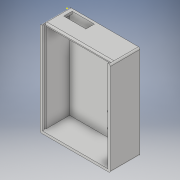
# Autodesk Inventor part: BatteryBox
Saved by Autodesk Inventor 2019 (Build 230136000, 136)
## iProperties
Created: 2018-06-02
Part Number: BatteryBox
Material: Generic
Document SubType Name: Modeling
Designer: samps
Density: 1 g/cm^3
Appearance: Default
Author: samps
Autodesk Inventor part; units mm, degrees
ref_plane "YZ Plane" through (0, 0, 0) normal (1, 0, 0) x (0, 1, 0)
ref_plane "XZ Plane" through (0, 0, 0) normal (0, 1, 0) x (-1, 0, 0)
ref_plane "XY Plane" through (0, 0, 0) normal (0, 0, 1) x (1, 0, 0)
sketch "Sketch1" plane through (0, 0, 0) normal (0, 0, 1) x (1, 0, 0)
  line L0 (0, 0) -> (90, 0)
  line L1 (90, 0) -> (90, -120)
  line L2 (90, -120) -> (0, -120)
  line L3 (0, -120) -> (0, 0)
  dimension "d0" = 90
  dimension "d1" = 120
  constraints: 8 end point, 2 parallel, 1 horizontal, 1 perpendicular
  measures "d0" distance of L1.end L2.end
  measures "d1" distance of L0.end L1.end
extrude "Extrusion1" add sketch "Sketch1" along normal blind 3.175
sketch "Sketch2" plane through (0, 0, 3.175) normal (0, 0, 1) x (1, 0, 0)
  point P0 (0, 0)
sketch "Sketch3" plane through (0, 0, 3.175) normal (0, 0, 1) x (1, 0, 0)
  line L0 (0, -120) -> (90, -120) projected
  line L1 (0, 0) -> (90, 0)
  line L2 (90, 0) -> (90, -120)
  line L3 (90, -120) -> (0, -120)
  line L4 (0, -120) -> (0, 0)
  line L5 (90, 0) -> (0, 0) projected
  line L6 (0, 0) -> (3.175, 0)
  line L7 (90, -120) -> (90, -116.825)
  line L8 (90, -120) -> (90, 0) projected
  line L9 (3.175, -3.175) -> (86.825, -3.175)
  line L10 (86.825, -3.175) -> (86.825, -116.825)
  line L11 (86.825, -116.825) -> (3.175, -116.825)
  line L12 (3.175, -116.825) -> (3.175, -3.175)
  dimension "d4" = 3.175
  dimension "d5" = 3.175
  dimension "d7" = 3.175
  constraints: 20 end point, 4 parallel, 2 horizontal, 2 perpendicular, 2 point on line
  measures "d4" distance of L1.start L6.end
  measures "d5" distance of L6.end L9.start
  measures "d7" distance of L7.end L10.end
extrude "Extrusion2" add sketch "Sketch3" along normal blind 30
sketch "Sketch4" plane through (0, 0, 33.175) normal (0, 0, 1) x (1, 0, 0)
  line L0 (0, 0) -> (90, 0) projected
  line L1 (0, -120) -> (0, 0) projected
  line L2 (0, 0) -> (0, -120)
  line L3 (90, -120) -> (0, -120) projected
  line L4 (0, -120) -> (90, -120)
  line L5 (90, -120) -> (90, 0)
  line L6 (90, 0) -> (88, 0)
  line L7 (88, 0) -> (88, -116.825)
  line L8 (3.175, -116.825) -> (86.825, -116.825) projected
  line L9 (88, -116.825) -> (3.175, -116.825)
  line L10 (3.175, -116.825) -> (2, -116.825)
  line L11 (2, -116.825) -> (2, 0)
  line L12 (2, 0) -> (0, 0)
  dimension "d10" = 2
  dimension "d11" = 1.175
  constraints: 18 end point, 5 perpendicular, 2 collinear, 2 point on line, 1 vertical
  measures "d10" distance of L5.end L6.end
  measures "d11" distance of L8.start L10.end
extrude "Extrusion3" add sketch "Sketch4" along normal blind 2.75 contours L0 L11 L10 L8 L9 L7 L5 L3 L1
sketch "Sketch5" plane through (0, 0, 35.925) normal (0, 0, 1) x (1, 0, 0)
  line L0 (0, 0) -> (90, 0) projected
  line L1 (0, 0) -> (3.175, 0)
  line L2 (86.825, -3.175) -> (3.175, -3.175) projected
  line L3 (3.175, -116.825) -> (86.825, -116.825) projected
  line L4 (3.175, 0) -> (3.175, -116.825)
  line L5 (3.175, -116.825) -> (86.825, -116.825)
  line L6 (86.825, -116.825) -> (86.825, 0)
  line L7 (90, 0) -> (90, -120) projected
  line L8 (86.825, 0) -> (90, 0)
  line L9 (90, 0) -> (90, -120)
  line L10 (90, -120) -> (0, -120) projected
  line L11 (90, -120) -> (0, -120)
  line L12 (0, -120) -> (0, 0) projected
  line L13 (0, -120) -> (0, 0)
  line L14 (0, 0) -> (3.175, 0)
  constraints: 18 end point, 6 perpendicular, 2 collinear, 1 parallel, 1 point on line
extrude "Extrusion4" add sketch "Sketch5" along normal blind 2 contours L0 L4 L3 L6 L7 L10 L12
sketch "Sketch6" plane through (0, 0, 0) normal (0, 1, 0) x (1, 0, 0)
  line L0 (3.175, -3.175) -> (86.825, -3.175) projected
  line L1 (3.175, -3.175) -> (3.175, -33.175) projected
  line L2 (86.825, -3.175) -> (3.175, -3.175)
  line L3 (3.175, -3.175) -> (45, -3.175)
  line L4 (45, -13.925) -> (6.3314, -13.925)
  line L5 (6.3314, -13.925) -> (34.8314, -13.925)
  line L6 (34.8314, -13.925) -> (34.8314, -3.175)
  line L7 (34.8314, -3.175) -> (6.3314, -3.175)
  line L8 (6.3314, -3.175) -> (6.3314, -13.925)
  point P0 (0, 0)
  dimension "d16" = 10.75
  dimension "d18" = 28.5
  dimension "d46" = 3.1564
  constraints: 14 end point, 3 horizontal, 2 parallel, 1 midpoint, 1 perpendicular, 1 point on line
  measures "d16" distance of L3.end L4.start
  measures "d18" distance of L7.end L6.end
  measures "d46" distance between parallel lines of L1 L8
extrude "Extrusion5" cut sketch "Sketch6" against normal blind 3.175
sketch "Sketch7" plane through (0, 0, 3.175) normal (0, 0, 1) x (1, 0, 0)
  line L0 (0, -120) -> (90, -120) projected
  line L1 (90, -120) -> (34.437, -120)
  line L2 (34.437, -120) -> (34.437, -75.55)
  line L3 (34.437, -75.55) -> (90, -75.55)
  line L4 (90, -75.55) -> (90, -120)
  line L5 (90, -120) -> (34.437, -120)
  line L6 (62.2185, -120) -> (62.2185, -97.575)
  dimension "d22" = 55.563
  dimension "d23" = 44.45
  dimension "d24" = 22.425
  constraints: 12 end point, 2 parallel, 1 collinear, 1 horizontal, 1 midpoint, 1 perpendicular, 1 vertical
  measures "d22" distance of L2.end L3.end
  measures "d23" distance of L1.end L2.end
  measures "d24" distance of L6.start L6.end
hole "Hole1" at (62.2185, -97.575, 3.175) direction (0, 0, -1) diameter 10 end through all
sketch "Sketch8" plane through (0, 0, 3.175) normal (0, 0, 1) x (1, 0, 0)
  circle A0 centre (62.2185, -97.575) radius 5 projected
  line L0 (62.2185, -97.575) -> (71.7185, -97.575)
  line L1 (71.7185, -97.575) -> (71.7185, -88.075)
  line L2 (71.7185, -88.075) -> (52.7185, -88.075)
  line L3 (52.7185, -88.075) -> (52.7185, -107.075)
  line L4 (52.7185, -107.075) -> (71.7185, -107.075)
  line L5 (71.7185, -107.075) -> (71.7185, -88.075)
  point P0 (0, 0)
  dimension "d32" = 9.5
  dimension "d33" = 9.5
  dimension "d34" = 19
  dimension "d35" = 19
  constraints: 12 end point, 2 horizontal, 2 parallel, 2 perpendicular
  measures "d32" distance of L0.start L0.end
  measures "d33" distance of L0.end L1.end
  measures "d34" distance of L4.end L3.end
  measures "d35" distance of L3.end L2.end
hole "Hole2" at (52.7185, -88.075, 3.175) at (71.7185, -88.075, 3.175) at (71.7185, -107.075, 3.175) at (52.7185, -107.075, 3.175) direction (0, 0, -1) diameter 3 end through all
fillet "Fillet1" radius 2 2 edges at (0, 0, 18.9625) (90, 0, 18.9625)
fillet "Fillet2" radius 2 2 edges at (0, -120, 18.9625) (90, -120, 18.9625)
fillet "Fillet3" radius 2 1 edges at (45, 0, 33.175)
body "Solid1"
